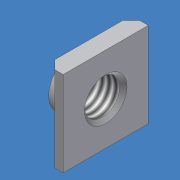
# Autodesk Inventor part: HNTTBS5-5
Saved by Autodesk Inventor 2014 SP1 (Build 180222100, 222)
## iProperties
Category: PARTsolutions
Created: 2015-02-04
Part Number: HNTTBS5-5
Catalog Web Link: www.cadenas.de
Description: HNTTBS - Nuts for Aluminum Frames Pre-Assembly Fitting Spring Nuts Standard Type
Document SubType Name: Modeling
Designer: PARTsolutions
Material: Generic
Density: 1 g/cm^3
Appearance: RGB(175,175,175)
NB: HNTTBS5-5
NN: HNTTBS
NT: Nuts for Aluminum Frames Pre-Assembly Fitting Spring Nuts Standard Type
NBSYN: $PN.
LINA: HNTTBS5-5
PN: HNTTBS5-5
TP: HNTTBS
MAT: 304 Stainless Steel
ST: -
NO: 5
M: 5
CFS: HFS5
CFSW: 6
CFT: 20, 40 sq.
MATT: '3','4','5'
A: 0.0
B: 10
E: 2
T: 3.7
L: 10
D: 6.7
MMIN: 4.134
MMAX: 5.000
TT: 6.8
MATALG: '304 Stainless Steel','304 Stainless Steel','1010 Steel (or Equivalent)','1010 Steel (or Equivalent)','316 Stainless Steel (or Equivalent)','316 Stainless Steel (or Equivalent)','303 Stainless Steel','303 Stainless Steel'
X: 0.7
D11: 6.000
KT: DUMMY
CreationOption_UseAsmMates: 0
SUPPLIER: Misumi
ARTICLENO: HNTTBS5-5
BOMINFO: HNTTBS5-5
CREATOR: CADENAS GmbH
PSOL_IDENT_0: {\\10.0.0.236\data_v8\23d-libs\misumi\metric\38_al_extrusions_blackets\nuts\hnttbs.prj},161 {VTYP=3D
PSOL_IDENT_1: },{NB=HNTTBS5-5},{LINA=HNTTBS5-5},{NN=HNTTBS},{DATE=19.11.2014 02:34:08},{GEOMDATE=17.09.2009 00:00:
PSOL_IDENT_2: 00},{VERSION=},{LINEID=20},{LINESUBID=-1},{WBVAR=M}  {NB=HNTTBS5-5},{LINA=HNTTBS5-5},{KT=DUMMY},{PN=
PSOL_IDENT_3: HNTTBS5-5},{TP=HNTTBS},{MAT=304 Stainless Steel},{ST=-},{NO=5},{M=5},{CFS=HFS5},{CFSW=6},{CFT=20, 40
PSOL_IDENT_4: sq.},{MATT='3','4','5'},{A=0.0},{B=10},{E=2},{T=3.7},{L=10},{D=6.7},{MMIN=4.134},{MMAX=5},{TT=6.8},
PSOL_IDENT_5: {MATALG='304 Stainless Steel','304 Stainless Steel','1010 Steel (or Equivalent)','1010 Steel (or Equ
PSOL_IDENT_6: ivalent)','316 Stainless Steel (or Equivalent)','316 Stainless Steel (or Equivalent)','303 Stainless
PSOL_IDENT_7: Steel','303 Stainless Steel'},{X=0.7},{D11=6}
Title: HNTTBS5-5
Author: Cadenas PARTsolutions
Comments: Nuts for Aluminum Frames Pre-Assembly Fitting Spring Nuts Standard Type
Autodesk Inventor part; units mm, degrees
sketch "Sketch_1" plane through (0, 0, 0) normal (0, 0, 1) x (1, 0, 0)
  line L0 (-2, -4) -> (-1, -5)
  line L1 (-1, -5) -> (0, -5)
  line L2 (0, -5) -> (0, 5)
  line L3 (0, 5) -> (-1, 5)
  line L4 (-1, 5) -> (-2, 4)
  line L5 (-2, 4) -> (-2, -4)
  constraints: 12 end point
extrude "Extrusion1" add sketch "Sketch_1" along normal mid plane 10
sketch "Sketch_10" plane through (0, 0, 0) normal (0, 0, 1) x (1, 0, 0)
  line L0 (-2, 0) -> (-3.7, 0)
  line L1 (-3.7, 0) -> (-3.7, 3)
  line L2 (-3.7, 3) -> (-2, 3.35)
  line L3 (-2, 3.35) -> (-2, 0)
  line L4 (-2, 0) -> (-3.7, 0)
  constraints: 10 end point
revolve "Revolution1" add sketch "Sketch_10" angle 360 about axis through (-2, 0, 0) along (1, 0, 0)
sketch "Sketch_3" plane through (0, 0, 0) normal (0, 0, 1) x (1, 0, 0)
  line L0 (0, 0) -> (-3.7, 0)
  line L1 (-3.7, 0) -> (-3.7, 2.5)
  line L2 (-3.7, 2.5) -> (-3.267, 2.067)
  line L3 (-3.267, 2.067) -> (-0.433, 2.067)
  line L4 (-0.433, 2.067) -> (0, 2.5)
  line L5 (0, 2.5) -> (0, 0)
  line L6 (0, 0) -> (-3.7, 0)
  constraints: 14 end point
revolve "Revolution2" cut sketch "Sketch_3" angle 360 about axis through (0, 0, 0) along (1, 0, 0)
thread "Thread1" size "M5x0.8" class "6H" standard "ISO Metric profile" full length
ref_plane "nut_XY" through (0, 0, 0) normal (1, 0, 0) x (0, 0, -1)
ref_plane "nut_YZ" through (0, 0, 0) normal (0, 0, -1) x (0, 1, 0)
ref_plane "nut_ZX" through (0, 0, 0) normal (0, 1, 0) x (1, 0, 0)
ref_plane "to_bolt_XY" through (-3.7, 0, 0) normal (1, 0, 0) x (0, 0, -1)
ref_plane "to_bolt_YZ" through (-3.7, 0, 0) normal (0, 0, -1) x (0, 1, 0)
ref_plane "to_bolt_ZX" through (-3.7, 0, 0) normal (0, 1, 0) x (1, 0, 0)
ref_plane "to_frames_XY" through (-2, 0, 0) normal (1, 0, 0) x (0, 0, -1)
ref_plane "to_frames_YZ" through (-2, 0, 0) normal (0, 0, -1) x (0, 1, 0)
ref_plane "to_frames_ZX" through (-2, 0, 0) normal (0, 1, 0) x (1, 0, 0)
body "Solid1"
